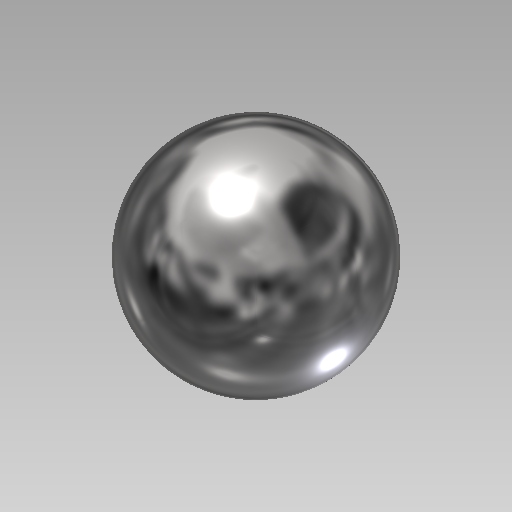
# Autodesk Inventor part: RF-1560ZZ_ball
Saved by Autodesk Inventor 2020 (Build 240168000, 168)
## iProperties
Created: 2019-10-06
Part Number: RF-1560ZZ_ball
Material: 鋼、炭素鋼
Catalog Web Link: www.cadenas.de
Description: Radial Flanged Ball Bearings (RF-Series/LF series) Metric ST ball-Radial Flanged Ball Bearings (RF-Series/LF series) Metric Shielded Type
Vendor: NMB
Document SubType Name: Modeling
Designer: psadmin
Manufacturer: NMB
Mass: 0.0881276 g
Surface Area: 0.242463 cm^2
Volume: 0.0112264 cm^3
Density: 7.85 g/cm^3
Appearance: 半つや出し
Category: PARTsolutions
Company: NMB
PSOL_IDENT_0: {$CADENAS_DATA\23d-libs\nmb\pbbp\radial_flanged_ball_bearings\rfbb_rflfs_m\rflf_shielded_ball.prj},2
PSOL_IDENT_1: 29 {VTYP=3D},{NB=RF-1560ZZ_ball},{LINA=RF-1560ZZ_ball},{NN=Radial Flanged Ball Bearings (RF-Series/L
PSOL_IDENT_2: F series) Metric ST ball},{DATE=11.11.2013 05:13:45},{GEOMDATE=24.10.2013 09:50:00},{VERSION=},{LINE
PSOL_IDENT_3: ID=1490},{WBVAR=},{WBNUMERIC=}  {NB=RF-1560ZZ_ball},{LINA=RF-1560ZZ_ball},{KT=DUMMY},{IDNR=},{PN=RF-
PSOL_IDENT_4: 1560ZZ},{SHLD=shielded},{FLANG=flanged},{SD=6.000},{D=15.000},{B=5.000},{SR=0.20},{BCZ=7},{DW=2.7781
PSOL_IDENT_5: },{LI=7.80},{LO=13.20},{D1=17.000},{C1=1.20},{D2=0.0},{C2=0.00},{COR=671},{CR=1058},{PCD=10.500},{U=
PSOL_IDENT_6: 13.278},{W=7.722},{Y=1.389},{Z=1.389},{AA=13.000},{AC=1.00},{AD=0.000},{AF=0.00},{AQ=0.20},{AH=13.40
PSOL_IDENT_7: },{AI=8.00},{AJ=0.40}
NN: Radial Flanged Ball Bearings (RF-Series/LF series) Metric ST ball
NT: Radial Flanged Ball Bearings (RF-Series/LF series) Metric Shielded Type
NB: RF-1560ZZ_ball
NBSYN: $PN._ball
LINA: RF-1560ZZ_ball
PN: RF-1560ZZ
SHLD: shielded
FLANG: flanged
SD: 6
D: 15
B: 5
SR: 0.2
BCZ: 7
DW: 2.7781
LI: 7.8
LO: 13.2
D1: 17
C1: 1.2
D2: 0
C2: 0
COR: 671
CR: 1058
PCD: 10.5
U: 13.278
W: 7.722
Y: 1.389
Z: 1.389
AA: 13
AC: 1
AD: 0
AF: 0
AQ: 0.2
AH: 13.4
AI: 8
AJ: 0.4
SUPPLIER: NMB
ARTICLENO: RF-1560ZZ_ball
BOMINFO: RF-1560ZZ_ball
CREATOR: CADENAS GmbH
Title: RF-1560ZZ_ball
Author: Cadenas PARTsolutions
Comments: Radial Flanged Ball Bearings (RF-Series/LF series) Metric Shielded Type
Autodesk Inventor part; units mm, degrees
sketch "Sketch_1" plane through (0, 0, 0) normal (0, 0, 1) x (1, 0, 0)
  line L0 (1.3891, 0) -> (-1.3891, 0)
  arc A0 (1.3891, 0) -> (-1.3891, 0) centre (0, 0) ccw
  line L1 (1.3891, 0) -> (-1.3891, 0)
  constraints: 4 end point, 2 point on circle, 1 centre point
revolve "Revolution1" add sketch "Sketch_1" angle 360 about axis through (1.3891, 0, 0) along (1, 0, 0)
ref_plane "1_XY" through (0, 0, 0) normal (0, 0, 1) x (1, 0, 0)
ref_plane "1_YZ" through (0, 0, 0) normal (1, 0, 0) x (0, 1, 0)
ref_plane "1_ZX" through (0, 0, 0) normal (0, 1, 0) x (0, 0, 1)
body "Solid1"
